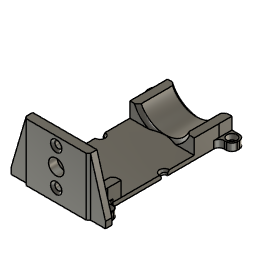
MotorHouder v7 (Autodesk Fusion 360 design; units mm, degrees)
Autodesk Fusion 360 part; units mm, degrees
sketch "Sketch1" plane through (0, 0, 0) normal (0, 0, 1) x (1, 0, 0)
  line L0 (0, 0) -> (30, 0)
  line L1 (30, 0) -> (30, 63)
  line L2 (30, 63) -> (0, 63)
  line L3 (0, 63) -> (0, 0)
  line L4 (0, 0) -> (30, 0)
  line L5 (30, 0) -> (30, -3)
  line L6 (30, -3) -> (0, -3)
  line L7 (0, -3) -> (0, 0)
  line L8 (0, -3) -> (-7, -3)
  line L9 (30, -3) -> (37, -3)
  line L10 (-7, -3) -> (0, -3)
  line L11 (0, -3) -> (0, 0)
  line L12 (0, 0) -> (-7, 0)
  line L13 (-7, 0) -> (-7, -3)
  line L14 (30, 0) -> (37, 0)
  line L15 (37, 0) -> (37, -3)
  line L16 (37, -3) -> (30, -3)
  line L17 (30, -3) -> (30, 0)
  line L18 (0, 63) -> (-6, 63)
  line L19 (-6, 63) -> (-6, 57)
  line L20 (-6, 57) -> (0, 57)
  line L21 (0, 57) -> (0, 63)
  line L22 (30, 63) -> (36, 63)
  line L23 (36, 63) -> (36, 57)
  line L24 (36, 57) -> (30, 57)
  line L25 (30, 57) -> (30, 63)
  circle A0 centre (-3, 60) radius 1.5
  circle A1 centre (33, 60) radius 1.5
  circle A2 centre (0, 31.5) radius 1.5
  circle A3 centre (30, 31.5) radius 1.5
  line L26 (0, 0) -> (-5, 0)
  line L27 (-5, 0) -> (-5, 5)
  line L28 (0, 5) -> (0, 0)
  line L29 (30, 0) -> (36, 0)
  line L30 (30, 5) -> (30, 0)
  line L31 (0, 5) -> (-5, 5)
  line L32 (30, 0) -> (35, 0)
  line L33 (35, 0) -> (35, 5)
  line L34 (35, 5) -> (30, 5)
  line L35 (30, 5) -> (30, 0)
  circle A4 centre (-2.5, 2.5) radius 1.5
  circle A5 centre (32.5, 2.5) radius 1.5
  line L36 (0, -3) -> (30, -3)
  line L37 (30, -3) -> (30, -4)
  line L38 (30, -4) -> (0, -4)
  line L39 (0, -4) -> (0, -3)
  dimension "d2" = 63
  dimension "d3" = 3
  dimension "d4" = 3
  dimension "d5" = 3
  dimension "d6" = 3
  dimension "d7" = 5
  dimension "d13" = 5
  dimension "d14" = 5
  dimension "d15" = 3
  dimension "d16" = 3
  constraint horizontal L0
  constraint vertical L1
  constraint horizontal L2
  constraint vertical L3
  constraint coincident L0.start L3.end
  constraint horizontal L4
  constraint vertical L5
  constraint horizontal L6
  constraint vertical L7
  constraint perpendicular L7 L8
  constraint perpendicular L5 L9
  constraint horizontal L10
  constraint vertical L11
  constraint horizontal L12
  constraint vertical L13
  constraint horizontal L14
  constraint vertical L15
  constraint horizontal L16
  constraint vertical L17
  constraint horizontal L18
  constraint vertical L19
  constraint horizontal L20
  constraint vertical L21
  constraint horizontal L22
  constraint vertical L23
  constraint horizontal L24
  constraint vertical L25
  constraint midpoint L3 A2.centre
  constraint midpoint L1 A3.centre
  constraint horizontal L26
  constraint vertical L27
  constraint vertical L28
  constraint horizontal L29
  constraint vertical L30
  constraint perpendicular L27 L31
  constraint horizontal L32
  constraint vertical L33
  constraint horizontal L34
  constraint vertical L35
  constraint horizontal L36
  constraint vertical L37
  constraint horizontal L38
  constraint vertical L39
  measures "d2" distance of L0.start L2.end
  measures "d3" diameter of A0
  measures "d4" diameter of A1
  measures "d5" diameter of A2
  measures "d6" diameter of A3
  measures "d7" distance of L0.start L26.end
  measures "d13" distance of L0.end L32.end
  measures "d14" distance of L0.end L30.start
  measures "d15" diameter of A4
  measures "d16" diameter of A5
extrude "Extrude1" add sketch "Sketch1" along normal blind 2 contours L0 L1 L2 L3 L4 L21 L25 A2 A3 L28 L30 L35 | L3 L12 L26 L27 L28 L31 | L0 L4 L5 L6 L7 L11 L17 L36 | L7 L8 L10 L11 L12 L13 L26 | L5 L9 L14 L15 L16 L17 L29 L32 | L1 L14 L29 L30 L32 L33 L34 L35 | L6 L36 L37 L38 L39 | L3 L18 L19 L20 L21 | L1 L22 L23 L24 L25
extrude "Extrude2" add sketch "Sketch1" along normal blind 27 contours L0 L4 L5 L6 L7 L11 L17 L36 | L7 L8 L10 L11 L12 L13 L26 | L5 L9 L14 L15 L16 L17 L29 L32 | L6 L36 L37 L38 L39
chamfer "Chamfer1" distance 7 distance2 24 2 edges at (-7, -1.5, 27) (37, -1.5, 27) measured on face at (10, -1, 27) measured on face at (10, -1, 27)
sketch "Sketch2" plane through (0, 0, 2) normal (0, 0, 1) x (-1, 0, 0)
  line L0 (5, 0) -> (-35, 0)
  line L1 (-35, 0) -> (-35, -5)
  line L2 (-35, -5) -> (-30, -5)
  line L3 (-30, -5) -> (-30, -30)
  arc A0 (-30, -33) -> (-30, -30) centre (-30, -31.5) ccw
  line L4 (-30, -33) -> (-30, -57)
  line L5 (-30, -57) -> (-36, -57)
  line L6 (-36, -57) -> (-36, -63)
  line L7 (-36, -63) -> (6, -63)
  line L8 (6, -63) -> (6, -57)
  line L9 (6, -57) -> (0, -57)
  line L10 (0, -57) -> (0, -33)
  arc A1 (0, -30) -> (0, -33) centre (0, -31.5) ccw
  line L11 (0, -30) -> (0, -5)
  line L12 (0, -5) -> (5, -5)
  line L13 (5, -5) -> (5, 0)
  circle A2 centre (-33, -60) radius 1.5
  circle A3 centre (2.5, -2.5) radius 1.5
  circle A4 centre (-32.5, -2.5) radius 1.5
  circle A5 centre (3, -60) radius 1.5
  line L14 (-35, 0) -> (-30, 0)
  line L15 (-30, 0) -> (-30, -5)
  line L16 (-30, -5) -> (-35, -5)
  line L17 (-35, -5) -> (-35, 0)
  line L18 (5, 0) -> (0, 0)
  line L19 (0, 0) -> (0, -5)
  line L20 (0, -5) -> (5, -5)
  line L21 (5, -5) -> (5, 0)
  line L22 (0, -57) -> (6, -57)
  line L23 (6, -57) -> (6, -63)
  line L24 (6, -63) -> (0, -63)
  line L25 (0, -63) -> (0, -57)
  line L26 (-36, -57) -> (-30, -57)
  line L27 (-30, -57) -> (-30, -63)
  line L28 (-30, -63) -> (-36, -63)
  line L29 (-36, -63) -> (-36, -57)
  constraint horizontal L14
  constraint vertical L15
  constraint horizontal L16
  constraint vertical L17
  constraint coincident L2.end L3.start
  constraint coincident L0.end L1.start
  constraint horizontal L18
  constraint vertical L19
  constraint horizontal L20
  constraint vertical L21
  constraint coincident L11.end L12.start
  constraint coincident L0.start L13.end
  constraint horizontal L22
  constraint vertical L23
  constraint horizontal L24
  constraint vertical L25
  constraint coincident L7.end L8.start
  constraint coincident L9.end L10.start
  constraint horizontal L26
  constraint vertical L27
  constraint horizontal L28
  constraint vertical L29
  constraint coincident L7 L27.end
  constraint coincident L5.end L6.start
extrude "Extrude3" add sketch "Sketch2" along normal blind 1.4 contours L0 L12 L13 L18 L19 L20 L21 | L0 L1 L2 L14 L15 L16 L17 | L7 L8 L9 L22 L23 L24 L25 | L5 L6 L7 L26 L27 L28 L29
chamfer "Chamfer2" distance 0.8 distance2 2 4 edges at (-1.6015, 59.4576, 3.4) (34.3985, 59.4576, 3.4) (33.8985, 1.9576, 3.4) (-1.1015, 1.9576, 3.4) measured on face at (-2.9626, 62.4986, 3.4) measured on face at (33.0374, 62.4986, 3.4) measured on face at (32.5374, 0.3347, 3.4) measured on face at (-2.5374, 4.6653, 3.4)
chamfer "Chamfer2" distance 0.8 distance2 1 2 edges at (1.5, 31.5, 2) (28.5, 31.5, 2) measured on face at (19.6599, 13.4668, 2) measured on face at (19.6599, 13.4668, 2)
sketch "Sketch3" plane through (0, 0, 0) normal (0, 1, 0) x (-1, 0, 0)
  line L0 (-30, 2) -> (0, 2)
  line L1 (0, 3.4) -> (5, 3.4)
  line L2 (5, 3.4) -> (5, 0)
  line L3 (5, 0) -> (7, 0)
  line L4 (7, 0) -> (7, 3)
  line L5 (7, 3) -> (0, 27)
  line L6 (0, 27) -> (-30, 27)
  line L7 (-30, 27) -> (-37, 3)
  line L8 (-37, 3) -> (-37, 0)
  line L9 (-37, 0) -> (-35, 0)
  line L10 (-35, 0) -> (-35, 3.4)
  line L11 (-35, 3.4) -> (-30, 3.4)
  line L12 (-30, 27) -> (0, 27)
  line L13 (0, 27) -> (0, 2)
  line L14 (0, 2) -> (-30, 2)
  line L15 (-30, 2) -> (-30, 27)
  circle A0 centre (-15, 14.5) radius 12.5
  circle A1 centre (-15, 14.5) radius 8.5
  circle A2 centre (-15, 23) radius 1.25
  circle A3 centre (-15, 6) radius 1.25
  circle A4 centre (-15, 14.5) radius 2
  line L16 (-27.5, 14.5) -> (-27.5, 27)
  line L17 (-2.5, 14.5) -> (-2.5, 27)
  line L18 (-30, 3.4) -> (-30, 2)
  line L19 (0, 2) -> (0, 3.4)
  dimension "d29" = 25
  dimension "d30" = 25
  dimension "d31" = 17
  dimension "d32" = 2.5
  dimension "d34" = 360
  dimension "d35" = 4
  constraint horizontal L12
  constraint vertical L13
  constraint horizontal L14
  constraint vertical L15
  constraint coincident L6.end L7.start
  constraint concentric A0 A1
  constraint coincident A1 A2.centre
  constraint concentric A1 A4
  constraint coincident A0 L16.start
  constraint coincident L12 L16.end
  constraint tangent A0 L16
  constraint perpendicular L12 L16
  constraint coincident A0 L17.start
  constraint coincident L12 L17.end
  constraint tangent A0 L17
  constraint perpendicular L12 L17
  measures "d29" distance of L6.end L0.start
  measures "d30" diameter of A0
  measures "d31" diameter of A1
  measures "d32" diameter of A2
  measures "d35" diameter of A4
extrude "Extrude4" cut sketch "Sketch3" against normal blind 7 contours A1 A2 | A1 A2 | A1 A3 | A1 A3 | A4
chamfer "Chamfer4" distance 1 distance2 1 2 edges at (16.1654, -4, 22.548) (16.1654, -4, 5.548) measured on face at (4.3333, -4, 13.8333) measured on face at (4.3333, -4, 13.8333)
sketch "Sketch5" plane through (0, 0, 2) normal (0, 0, 1) x (-1, 0, 0)
  line L0 (-30, -63) -> (0, -63)
  line L1 (0, -57) -> (0, -33.8)
  line L2 (0, -29.2) -> (0, -5)
  line L3 (0, 0) -> (-30, 0)
  line L4 (-30, -5) -> (-30, -29.2)
  line L5 (-30, -33.8) -> (-30, -57)
  line L6 (-30, -45.4) -> (0, -45.4)
  line L7 (-30, -11.25) -> (0, -11.25)
  arc A0 (-30, -33.8) -> (-30, -29.2) centre (-30, -31.5) ccw
  arc A1 (0, -29.2) -> (0, -33.8) centre (0, -31.5) ccw
  line L8 (-30, -57) -> (-30, -63)
  line L9 (0, -63) -> (0, -57)
  line L10 (0, -5) -> (0, 0)
  line L11 (-30, 0) -> (-30, -5)
  constraint midpoint L5 L6.start
  constraint midpoint L1 L6.end
  constraint coincident L2 L7.end
  constraint perpendicular L2 L7
extrude "Extrude5" add sketch "Sketch5" along normal blind 7 contours L0 L1 L5 L6 L8 L9 | L2 L3 L4 L7 L10 L11
cylinder "CylinderPrimitive1" cut diameter 25 height 64 placed x (1, 0, 0) y (0, 0, -1) z (0, 1, 0) at (15, 0, 14.5)
fillet "Fillet1" radius 2.5 11 edges at (36, 63, 1.7) (36, 57, 1.7) (30, 57, 1.7) (-6, 63, 1.7) (0, 57, 1.7) (-6, 57, 1.7) (-5, 5, 1.7) (0, 5, 1.7) (35, 5, 1.7) (30, 5, 1) (30, 5, 2.7)
fillet "Fillet2" radius 3.5 2 edges at (-5, 0, 1.7) (35, 0, 1.7)
chamfer "Chamfer5" distance 1 distance2 1 2 edges at (0, -4, 13.5) (30, -4, 13.5) measured on face at (0, -3.6667, 9) measured on face at (4.3333, -4, 13.8333)
fillet "Fillet3" radius 1.5 tangency weight 0.18429 6 edges at (8.3856, 11.25, 3.8934) (21.6144, 11.25, 3.8934) (8.3856, 45.4, 3.8934) (21.6144, 45.4, 3.8934) (8.3856, 63, 3.8934) (21.6144, 63, 3.8934)
move_face "OffsetFaces2" offset -1.6 1 faces at (13.0099, -1.3333, 14.3009)
move_face "OffsetFaces3" offset -0.4 2 faces at (16.2252, -2, 23.2477) (13.7562, -1, 6.1245)
